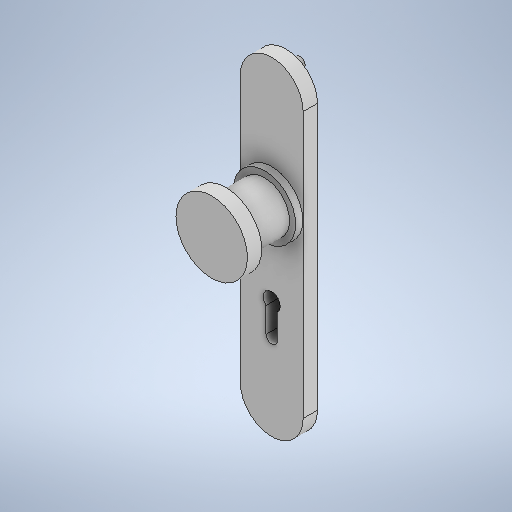
# Autodesk Inventor part: garnitur_rund
Saved by Autodesk Inventor 2025.1 (Build 291241000, 241)
## iProperties
Created: 2024-08-07
Part Number: garnitur_rund
Material: Generisch
Document SubType Name: Modeling
Designer: ffogue
Density: 1 g/cm^3
Appearance: Vorgabe
Author: ffogue
Autodesk Inventor part; units mm, degrees
ref_plane "YZ Plane" through (0, 0, 0) normal (1, 0, 0) x (0, 1, 0)
ref_plane "XZ Plane" through (0, 0, 0) normal (0, 1, 0) x (-1, 0, 0)
ref_plane "XY Plane" through (0, 0, 0) normal (0, 0, 1) x (1, 0, 0)
sketch "Sketch1" plane through (0, 0, 0) normal (0, 0, 1) x (1, 0, 0)
  line L0 (0, 0) -> (0, 42)
  line L1 (17.5, 37) -> (17.5, 10)
  line L2 (17.5, 10) -> (25, 10)
  line L3 (25, 10) -> (25, 0)
  line L4 (25, 0) -> (0, 0)
  line L5 (17.5, 37) -> (21.75, 37)
  line L6 (21.75, 37) -> (21.75, 42)
  line L7 (21.75, 42) -> (0, 42)
  dimension "d1" = 50
  dimension "d3" = 10
  dimension "d4" = 35
  dimension "d12" = 37
  dimension "d13" = 5
  dimension "d14" = 43.5
  constraints: 16 end point, 4 perpendicular, 2 vertical, 1 horizontal
  measures "d1" diameter of L3 L0
  measures "d3" distance between parallel lines of L4 L2
  measures "d4" diameter of L1 L0
  measures "d12" distance between parallel lines of L5 L4
  measures "d13" distance of L5.end L6.end
  measures "d14" diameter of L6 L0
revolve "Revolution1" add sketch "Sketch1" angle 360 about axis through (0, 0, 0) along (0, 1, 0)
sketch "Sketch3" plane through (0, 42, 0) normal (0, 1, 0) x (1, 0, 0)
  line L0 (0, -66) -> (0, 120) construction
  line L1 (-22, -66) -> (-22, 120)
  line L2 (22, 120) -> (22, -66)
  arc A0 (-22, -66) -> (22, -66) centre (0, -66) ccw
  arc A1 (22, 120) -> (-22, 120) centre (0, 120) ccw
  point P0 (0, 0)
  point P1 (0, 27)
  point P2 (0, -88)
  point P3 (0, 142)
  dimension "d16" = 44
  dimension "d17" = 88
  dimension "d18" = 230
  constraints: 8 end point, 6 point on circle, 4 tangent, 2 centre point, 1 midpoint, 1 parallel, 1 vertical, 1 vertical alignment
  measures "d16" distance between parallel lines of L1 L2
  measures "d17" distance of point (0, -88) point (0, 0)
  measures "d18" distance of point (0, 142) point (0, -88)
extrude "Extrusion2" add sketch "Sketch3" along normal blind 10
fillet "Fillet2" radius 2 1 edges at (-17.5, 10, 0)
sketch "Sketch4" plane through (0, 52, 0) normal (0, 1, 0) x (1, 0, 0)
  circle A0 centre (0, -75) radius 3.5
  circle A1 centre (0, 21.5) radius 3.5
  circle A2 centre (0, 112) radius 3.5
  circle A3 centre (0, 0) radius 21.75 projected
  point P0 (0, 0)
  dimension "d23" = 7
  dimension "d24" = 21.5
  dimension "d25" = 90.5
  dimension "d26" = 75
  constraints: 3 centre point, 3 vertical alignment, 2 equal radius
  measures "d23" diameter of A0
  measures "d24" distance of A1.centre point (0, 0)
  measures "d25" distance of A1.centre A2.centre
  measures "d26" distance of A0.centre point (0, 0)
extrude "Extrusion3" add sketch "Sketch4" along normal blind 10 contours A0 | A1 A3 | A3 A1 | A2 picked at (0.1355, 22.8044) picked at (-0.1398, 20.4874)
sketch "Sketch5" plane through (0, 42, 0) normal (0, -1, 0) x (1, 0, 0)
  arc A0 (4, -64.4721) -> (-4, -64.4721) centre (0, -60) ccw
  circle A1 centre (0, 0) radius 21.75 projected
  circle A2 centre (0, -112) radius 3.5 projected
  line L0 (-4, -64.4721) -> (-4, -82)
  arc A3 (-4, -82) -> (4, -82) centre (0, -82) ccw
  line L1 (4, -82) -> (4, -64.4721)
  dimension "d29" = 60
  dimension "d30" = 12
  dimension "d31" = 4
  dimension "d32" = 22
  constraints: 4 end point, 4 point on circle, 2 centre point, 2 vertical alignment, 1 horizontal alignment, 1 parallel, 1 tangent, 1 vertical
  measures "d29" distance of A0.centre A1.centre
  measures "d30" diameter of A0
  measures "d31" radius of A3
  measures "d32" distance of A3.centre A0.centre
extrude "Extrusion4" cut sketch "Sketch5" against normal blind 10 contours L1 A3 L0 A0
body "Solid1"
